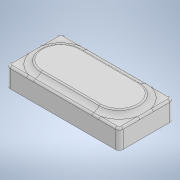
# Autodesk Inventor part: Keyboard Button
Saved by Autodesk Inventor 2021 (Build 250183000, 183)
## iProperties
Created: 2020-06-05
Part Number: Keyboard Button
Material: Generic
Document SubType Name: Modeling
Designer: ameli
Density: 1 g/cm^3
Appearance: Default
Author: ameli
Autodesk Inventor part; units mm, degrees
ref_plane "YZ Plane" through (0, 0, 0) normal (1, 0, 0) x (0, 1, 0)
ref_plane "XZ Plane" through (0, 0, 0) normal (0, 1, 0) x (-1, 0, 0)
ref_plane "XY Plane" through (0, 0, 0) normal (0, 0, 1) x (1, 0, 0)
sketch "Sketch1" plane through (0, 0, 0) normal (0, 1, 0) x (-1, 0, 0)
  line L0 (14.5, 7) -> (-14.5, 7)
  line L1 (-14.5, 7) -> (-14.5, -7)
  line L2 (-14.5, -7) -> (14.5, -7)
  line L3 (14.5, -7) -> (14.5, 7)
  point P0 (0, 0)
  dimension "d0" = 29
  dimension "d1" = 14
  dimension "d2" = 7
  dimension "d3" = 14.5
  constraints: 8 end point, 2 parallel, 1 horizontal, 1 perpendicular
  measures "d0" distance of L1.end L2.end
  measures "d1" distance of L0.end L1.end
  measures "d2" distance from line of point (0, 0) L2
  measures "d3" distance from line of point (0, 0) L3
extrude "Extrusion1" add sketch "Sketch1" along normal blind 5
sketch "Sketch2" plane through (0, 5, 0) normal (0, 1, 0) x (1, 0, 0)
  circle A0 centre (-7.5, 0) radius 5
  circle A1 centre (7.5, 0) radius 5
  line L0 (-14.5, 7) -> (-14.5, -7) projected
  line L1 (14.5, 7) -> (-14.5, 7) projected
  line L2 (14.5, -7) -> (14.5, 7) projected
  line L3 (-7.5, -5) -> (7.5, -5)
  line L4 (-7.5, 5) -> (7.5, 5)
  point P0 (0, 0)
  dimension "d6" = 10
  dimension "d7" = 10
  dimension "d8" = 7
  dimension "d9" = 7
  dimension "d10" = 7
  dimension "d11" = 7
  dimension "d12" = 5
  dimension "d13" = 5
  constraints: 4 end point, 4 point on circle, 2 centre point, 2 horizontal
  measures "d6" diameter of A0
  measures "d7" diameter of A1
  measures "d8" distance from line of L0 A0.centre
  measures "d9" distance from line of L1 A0.centre
  measures "d10" distance from line of L1 A1.centre
  measures "d11" distance from line of L2 A1.centre
  measures "d12" distance from line of point (0, 0) L3
  measures "d13" distance from line of point (0, 0) L4
extrude "Extrusion2" add sketch "Sketch2" along normal blind 1
fillet "Fillet1" radius 2 4 edges at (-12.5, 5, 0) (0, 5, -5) (12.5, 5, 0) (0, 5, 5)
fillet "Fillet2" radius 1 4 edges at (14.5, 2.5, 7) (14.5, 2.5, -7) (-14.5, 2.5, -7) (-14.5, 2.5, 7)
fillet "Fillet3" radius 0.5 12 edges at (14.2071, 5, 6.7071) (14.5, 5, 0) (14.2071, 5, -6.7071) (0, 5, -7) (-14.2071, 5, -6.7071) (-14.5, 5, 0) (-14.2071, 5, 6.7071) (0, 5, 7) (0, 6, -5) (-12.5, 6, 0) (0, 6, 5) (12.5, 6, 0)
sketch "Sketch5" plane through (0, 0, 0) normal (0, -1, 0) x (1, 0, 0)
  line L0 (10.5, 3) -> (-10.5, 3)
  line L1 (-10.5, 3) -> (-10.5, -3)
  line L2 (-10.5, -3) -> (10.5, -3)
  line L3 (10.5, -3) -> (10.5, 3)
  line L4 (14.5, 6) -> (14.5, -6) projected
  line L5 (13.5, -7) -> (-13.5, -7) projected
  line L6 (-13.5, 7) -> (13.5, 7) projected
  line L7 (-14.5, -6) -> (-14.5, 6) projected
  point P0 (0, 0)
  dimension "d37" = 4
  dimension "d38" = 4
  dimension "d39" = 4
  dimension "d40" = 4
  constraints: 8 end point, 2 parallel, 1 horizontal, 1 perpendicular
  measures "d37" distance between parallel lines of L4 L3
  measures "d38" distance between parallel lines of L5 L2
  measures "d39" distance between parallel lines of L6 L0
  measures "d40" distance between parallel lines of L7 L1
extrude "Extrusion6" cut sketch "Sketch5" against normal blind 4.5
body "Solid1"
